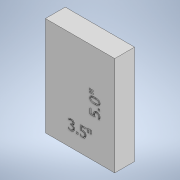
# Autodesk Inventor part: rectangular3_5x5_0-in-Template
Saved by Autodesk Inventor 2020.2 (Build 242310000, 310)
## iProperties
Created: 2020-01-27
Part Number: rectangular3_5x5_0-in-Template
Material: Generic
Document SubType Name: Modeling
Designer: robst
Density: 1 g/cm^3
Appearance: Default
Author: robst
Autodesk Inventor part; units mm, degrees
ref_plane "YZ Plane" through (0, 0, 0) normal (1, 0, 0) x (0, 1, 0)
ref_plane "XZ Plane" through (0, 0, 0) normal (0, 1, 0) x (-1, 0, 0)
ref_plane "XY Plane" through (0, 0, 0) normal (0, 0, 1) x (1, 0, 0)
sketch "Sketch1" plane through (0, 0, 0) normal (0, 0, 1) x (1, 0, 0)
  line L0 (-44.45, -63.5) -> (44.45, -63.5)
  line L1 (44.45, -63.5) -> (44.45, 63.5)
  line L2 (44.45, 63.5) -> (-44.45, 63.5)
  line L3 (-44.45, 63.5) -> (-44.45, -63.5)
  line L4 (-44.45, -63.5) -> (44.45, 63.5) construction
  line L5 (44.45, -63.5) -> (-44.45, 63.5) construction
  point P0 (0, 0)
  dimension "d0" = 88.9
  dimension "d1" = 127
  constraints: 12 end point, 2 midpoint, 2 parallel, 1 horizontal, 1 perpendicular
  measures "d0" distance of L0.start L0.end
  measures "d1" distance of L1.end L0.end
extrude "Extrusion1" add sketch "Sketch1" along normal mid plane 25.4
sketch "Sketch2" plane through (0, 0, 12.7) normal (0, 0, 1) x (1, 0, 0)
  line L0 (-44.45, 63.5) -> (-44.45, -63.5) construction
  line L1 (-44.45, -38.1) -> (44.45, -38.1) construction
  line L2 (44.45, -63.5) -> (44.45, 63.5) construction
  line L3 (-44.45, -63.5) -> (44.45, -63.5) construction
  line L4 (19.05, -63.5) -> (19.05, 63.5) construction
  spline S0 degree 2 poles (21.3656, -7.055) (22.2816, -7.055) (23.8459, -7.6416) (24.4223, -8.1768) knots 0 0 0 1 2 2 2
  spline S1 degree 2 poles (24.4223, -8.1768) (24.9986, -8.712) (25.6676, -10.3072) (25.6676, -11.2952) knots 0 0 0 1 2 2 2
  spline S2 degree 2 poles (25.6676, -11.2952) (25.6676, -12.2008) (25.2662, -13.971) (24.9472, -14.6194) knots 0 0 0 1 2 2 2
  line L5 (24.9472, -14.6194) -> (23.1461, -14.6194)
  line L6 (23.1461, -14.6194) -> (23.1461, -14.4959)
  spline S3 degree 2 poles (23.1461, -14.4959) (23.2902, -14.3004) (23.6607, -13.5697) (23.8254, -13.1271) knots 0 0 0 1 2 2 2
  spline S4 degree 2 poles (23.8254, -13.1271) (24.0003, -12.6228) (24.1959, -11.7892) (24.1959, -11.2643) knots 0 0 0 1 2 2 2
  spline S5 degree 2 poles (24.1959, -11.2643) (24.1959, -10.7497) (23.8254, -9.7823) (23.424, -9.4324) knots 0 0 0 1 2 2 2
  spline S6 degree 2 poles (23.424, -9.4324) (23.0432, -9.1133) (22.0346, -8.784) (21.3553, -8.784) knots 0 0 0 1 2 2 2
  spline S7 degree 2 poles (21.3553, -8.784) (20.6761, -8.784) (19.8116, -9.1545) (19.5234, -9.5044) knots 0 0 0 1 2 2 2
  spline S8 degree 2 poles (19.5234, -9.5044) (19.2044, -9.8646) (18.9368, -10.935) (18.9368, -11.5833) knots 0 0 0 1 2 2 2
  spline S9 degree 2 poles (18.9368, -11.5833) (18.9368, -12.2832) (19.1529, -13.6726) (19.2455, -14.0945) knots 0 0 0 1 2 2 2
  line L7 (19.2455, -14.0945) -> (12.7, -14.0945)
  line L8 (12.7, -14.0945) -> (12.7, -7.127)
  line L9 (12.7, -7.127) -> (14.1923, -7.127)
  line L10 (14.1923, -7.127) -> (14.1923, -12.4581)
  line L11 (14.1923, -12.4581) -> (17.5783, -12.4581)
  spline S10 degree 2 poles (17.5783, -12.4581) (17.5371, -12.1494) (17.5062, -11.5525) (17.5062, -11.3055) knots 0 0 0 1 2 2 2
  spline S11 degree 2 poles (17.5062, -11.3055) (17.5062, -10.3278) (17.8253, -8.9795) (18.2987, -8.362) knots 0 0 0 1 2 2 2
  spline S12 degree 2 poles (18.2987, -8.362) (18.7721, -7.7342) (20.213, -7.055) (21.3656, -7.055) knots 0 0 0 1 2 2 2
  line L12 (25.4, -2.4957) -> (25.4, -4.5335)
  line L13 (25.4, -4.5335) -> (22.9712, -4.5335)
  line L14 (22.9712, -4.5335) -> (22.9712, -2.4957)
  line L15 (22.9712, -2.4957) -> (25.4, -2.4957)
  spline S13 degree 2 poles (19.05, 7.9709) (22.4669, 7.9709) (25.6676, 5.9846) (25.6676, 3.916) knots 0 0 0 1 2 2 2
  spline S14 degree 2 poles (25.6676, 3.916) (25.6676, 1.8165) (22.4051, -0.1492) (19.0603, -0.1492) knots 0 0 0 1 2 2 2
  spline S15 degree 2 poles (19.0603, -0.1492) (15.6229, -0.1492) (12.4427, 1.8371) (12.4427, 3.916) knots 0 0 0 1 2 2 2
  spline S16 degree 2 poles (12.4427, 3.916) (12.4427, 6.0052) (15.7361, 7.9709) (19.05, 7.9709) knots 0 0 0 1 2 2 2
  spline S17 degree 2 poles (22.9197, 5.7891) (22.2919, 6.0361) (20.3571, 6.2419) (19.05, 6.2419) knots 0 0 0 1 2 2 2
  spline S18 degree 2 poles (19.05, 6.2419) (17.7429, 6.2419) (15.8184, 6.0361) (15.17, 5.7788) knots 0 0 0 1 2 2 2
  spline S19 degree 2 poles (15.17, 5.7788) (14.5216, 5.5215) (13.8527, 4.6261) (13.8527, 3.916) knots 0 0 0 1 2 2 2
  spline S20 degree 2 poles (13.8527, 3.916) (13.8527, 3.2059) (14.5216, 2.2899) (15.1906, 2.0223) knots 0 0 0 1 2 2 2
  spline S21 degree 2 poles (15.1906, 2.0223) (15.839, 1.765) (17.815, 1.5798) (19.0603, 1.5798) knots 0 0 0 1 2 2 2
  spline S22 degree 2 poles (19.0603, 1.5798) (20.3982, 1.5798) (22.189, 1.7444) (22.8888, 2.012) knots 0 0 0 1 2 2 2
  spline S23 degree 2 poles (22.8888, 2.012) (23.5475, 2.259) (24.2576, 3.175) (24.2576, 3.916) knots 0 0 0 1 2 2 2
  spline S24 degree 2 poles (24.2576, 3.916) (24.2576, 4.6158) (23.5887, 5.5318) (22.9197, 5.7891) knots 0 0 0 1 2 2 2
  line L16 (12.134, 11.501) -> (17.074, 11.1305)
  line L17 (17.074, 11.1305) -> (17.074, 10.0087)
  line L18 (17.074, 10.0087) -> (12.134, 9.6382)
  line L19 (12.134, 9.6382) -> (12.134, 11.501)
  line L20 (12.134, 14.712) -> (17.074, 14.3415)
  line L21 (17.074, 14.3415) -> (17.074, 13.2197)
  line L22 (17.074, 13.2197) -> (12.134, 12.8492)
  line L23 (12.134, 12.8492) -> (12.134, 14.712)
  spline S25 degree 2 poles (-11.3261, -32.9541) (-11.7892, -32.9541) (-12.7051, -33.1806) (-13.1477, -33.3555) knots 0 0 0 1 2 2 2
  spline S26 degree 2 poles (-13.1477, -33.3555) (-13.5594, -33.5305) (-14.1666, -33.901) (-14.4033, -34.0656) knots 0 0 0 1 2 2 2
  line L24 (-14.4033, -34.0656) -> (-14.5062, -34.0656)
  line L25 (-14.5062, -34.0656) -> (-14.5062, -32.2646)
  spline S27 degree 2 poles (-14.5062, -32.2646) (-13.9504, -31.9661) (-12.0465, -31.4824) (-11.1923, -31.4824) knots 0 0 0 1 2 2 2
  spline S28 degree 2 poles (-11.1923, -31.4824) (-10.3278, -31.4824) (-9.0413, -31.8323) (-8.5164, -32.2028) knots 0 0 0 1 2 2 2
  spline S29 degree 2 poles (-8.5164, -32.2028) (-7.9607, -32.6042) (-7.3843, -33.7672) (-7.3843, -34.5494) knots 0 0 0 1 2 2 2
  spline S30 degree 2 poles (-7.3843, -34.5494) (-7.3843, -35.5991) (-8.7634, -37.184) (-9.7308, -37.3899) knots 0 0 0 1 2 2 2
  line L26 (-9.7308, -37.3899) -> (-9.7308, -37.5134)
  spline S31 degree 2 poles (-9.7308, -37.5134) (-9.3295, -37.5957) (-8.4135, -37.9662) (-8.0224, -38.3367) knots 0 0 0 1 2 2 2
  spline S32 degree 2 poles (-8.0224, -38.3367) (-7.6313, -38.6969) (-7.1373, -39.8496) (-7.1373, -40.6832) knots 0 0 0 1 2 2 2
  spline S33 degree 2 poles (-7.1373, -40.6832) (-7.1373, -41.5374) (-7.7239, -42.9886) (-8.2591, -43.5443) knots 0 0 0 1 2 2 2
  spline S34 degree 2 poles (-8.2591, -43.5443) (-8.8149, -44.1207) (-10.3895, -44.7176) (-11.3878, -44.7176) knots 0 0 0 1 2 2 2
  spline S35 degree 2 poles (-11.3878, -44.7176) (-12.3449, -44.7176) (-14.218, -44.2545) (-14.8561, -43.9354) knots 0 0 0 1 2 2 2
  line L27 (-14.8561, -43.9354) -> (-14.8561, -42.1344)
  line L28 (-14.8561, -42.1344) -> (-14.7326, -42.1344)
  spline S36 degree 2 poles (-14.7326, -42.1344) (-14.1974, -42.5254) (-12.3861, -43.2459) (-11.4907, -43.2459) knots 0 0 0 1 2 2 2
  spline S37 degree 2 poles (-11.4907, -43.2459) (-10.9658, -43.2459) (-9.9161, -42.9165) (-9.5662, -42.5357) knots 0 0 0 1 2 2 2
  spline S38 degree 2 poles (-9.5662, -42.5357) (-9.2265, -42.1549) (-8.8663, -41.2493) (-8.8663, -40.5597) knots 0 0 0 1 2 2 2
  spline S39 degree 2 poles (-8.8663, -40.5597) (-8.8663, -39.8702) (-9.2677, -38.9748) (-9.6279, -38.7175) knots 0 0 0 1 2 2 2
  spline S40 degree 2 poles (-9.6279, -38.7175) (-9.9881, -38.4602) (-10.9658, -38.2647) (-11.5422, -38.2647) knots 0 0 0 1 2 2 2
  line L29 (-11.5422, -38.2647) -> (-12.2626, -38.2647)
  line L30 (-12.2626, -38.2647) -> (-12.2626, -36.8547)
  line L31 (-12.2626, -36.8547) -> (-11.6966, -36.8547)
  spline S41 degree 2 poles (-11.6966, -36.8547) (-10.5542, -36.8547) (-9.1133, -35.7638) (-9.1133, -34.7243) knots 0 0 0 1 2 2 2
  spline S42 degree 2 poles (-9.1133, -34.7243) (-9.1133, -34.2406) (-9.4838, -33.5511) (-9.7823, -33.3452) knots 0 0 0 1 2 2 2
  spline S43 degree 2 poles (-9.7823, -33.3452) (-10.1013, -33.1291) (-10.8835, -32.9541) (-11.3261, -32.9541) knots 0 0 0 1 2 2 2
  line L32 (-2.4957, -44.45) -> (-4.5335, -44.45)
  line L33 (-4.5335, -44.45) -> (-4.5335, -42.0212)
  line L34 (-4.5335, -42.0212) -> (-2.4957, -42.0212)
  line L35 (-2.4957, -42.0212) -> (-2.4957, -44.45)
  spline S44 degree 2 poles (7.7651, -40.4156) (7.7651, -41.3316) (7.1785, -42.8959) (6.6433, -43.4723) knots 0 0 0 1 2 2 2
  spline S45 degree 2 poles (6.6433, -43.4723) (6.1081, -44.0486) (4.5129, -44.7176) (3.5249, -44.7176) knots 0 0 0 1 2 2 2
  spline S46 degree 2 poles (3.5249, -44.7176) (2.6192, -44.7176) (0.8491, -44.3162) (0.2007, -43.9972) knots 0 0 0 1 2 2 2
  line L36 (0.2007, -43.9972) -> (0.2007, -42.1961)
  line L37 (0.2007, -42.1961) -> (0.3242, -42.1961)
  spline S47 degree 2 poles (0.3242, -42.1961) (0.5197, -42.3402) (1.2504, -42.7107) (1.693, -42.8754) knots 0 0 0 1 2 2 2
  spline S48 degree 2 poles (1.693, -42.8754) (2.1973, -43.0503) (3.0309, -43.2459) (3.5558, -43.2459) knots 0 0 0 1 2 2 2
  spline S49 degree 2 poles (3.5558, -43.2459) (4.0704, -43.2459) (5.0378, -42.8754) (5.3877, -42.474) knots 0 0 0 1 2 2 2
  spline S50 degree 2 poles (5.3877, -42.474) (5.7068, -42.0932) (6.0361, -41.0846) (6.0361, -40.4053) knots 0 0 0 1 2 2 2
  spline S51 degree 2 poles (6.0361, -40.4053) (6.0361, -39.7261) (5.6656, -38.8616) (5.3157, -38.5734) knots 0 0 0 1 2 2 2
  spline S52 degree 2 poles (5.3157, -38.5734) (4.9555, -38.2544) (3.8851, -37.9868) (3.2368, -37.9868) knots 0 0 0 1 2 2 2
  spline S53 degree 2 poles (3.2368, -37.9868) (2.5369, -37.9868) (1.1475, -38.2029) (0.7256, -38.2955) knots 0 0 0 1 2 2 2
  line L38 (0.7256, -38.2955) -> (0.7256, -31.75)
  line L39 (0.7256, -31.75) -> (7.6931, -31.75)
  line L40 (7.6931, -31.75) -> (7.6931, -33.2423)
  line L41 (7.6931, -33.2423) -> (2.362, -33.2423)
  line L42 (2.362, -33.2423) -> (2.362, -36.6283)
  spline S54 degree 2 poles (2.362, -36.6283) (2.6707, -36.5871) (3.2676, -36.5562) (3.5146, -36.5562) knots 0 0 0 1 2 2 2
  spline S55 degree 2 poles (3.5146, -36.5562) (4.4923, -36.5562) (5.8406, -36.8753) (6.4581, -37.3487) knots 0 0 0 1 2 2 2
  spline S56 degree 2 poles (6.4581, -37.3487) (7.0859, -37.8221) (7.7651, -39.263) (7.7651, -40.4156) knots 0 0 0 1 2 2 2
  line L43 (11.501, -31.184) -> (11.1305, -36.124)
  line L44 (11.1305, -36.124) -> (10.0087, -36.124)
  line L45 (10.0087, -36.124) -> (9.6382, -31.184)
  line L46 (9.6382, -31.184) -> (11.501, -31.184)
  line L47 (14.712, -31.184) -> (14.3415, -36.124)
  line L48 (14.3415, -36.124) -> (13.2197, -36.124)
  line L49 (13.2197, -36.124) -> (12.8492, -31.184)
  line L50 (12.8492, -31.184) -> (14.712, -31.184)
  point P0 (0, 0)
  dimension "d4" = 25.4
  dimension "d5" = 25.4
  constraints: 4 end point, 3 point on line, 2 horizontal, 2 vertical
  measures "d4" distance between parallel lines of L1 L3
  measures "d5" distance between parallel lines of L4 L2
extrude "Extrusion2" cut sketch "Sketch2" against normal blind 2.54
body "Solid1"
